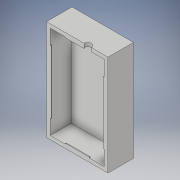
# Autodesk Inventor part: feeder_encolsure
Saved by Autodesk Inventor 2019 (Build 230136000, 136)
## iProperties
Created: 2018-11-21
Part Number: feeder_encolsure
Material: Generic
Document SubType Name: Modeling
Designer: chill
Density: 1 g/cm^3
Appearance: Default
Author: chill
Autodesk Inventor part; units mm, degrees
ref_plane "YZ Plane" through (0, 0, 0) normal (1, 0, 0) x (0, 1, 0)
ref_plane "XZ Plane" through (0, 0, 0) normal (0, 1, 0) x (-1, 0, 0)
ref_plane "XY Plane" through (0, 0, 0) normal (0, 0, 1) x (1, 0, 0)
sketch "Sketch1" plane through (0, 0, 0) normal (0, 0, 1) x (1, 0, 0)
  line L0 (0, 0) -> (36, 0)
  line L1 (36, 0) -> (36, 62)
  line L2 (36, 62) -> (0, 62)
  line L3 (0, 62) -> (0, 0)
  line L4 (-2.5, -2.5) -> (38.5, -2.5)
  line L5 (38.5, -2.5) -> (38.5, 64.5)
  line L6 (38.5, 64.5) -> (-2.5, 64.5)
  line L7 (-2.5, 64.5) -> (-2.5, -2.5)
  dimension "d0" = 36
  dimension "d1" = 62
  dimension "d2" = 2.5
  constraints: 16 end point, 4 parallel, 2 perpendicular, 1 horizontal, 3 other
  measures "d0" distance of L2.end L1.end
  measures "d1" distance of L1.end L0.end
  measures "d2" distance between parallel lines of L3 L7
extrude "Extrusion1" add sketch "Sketch1" along normal blind 17 contours L3 L2 L1 L0 | L7 L6 L5 L4
sketch "Sketch2" plane through (0, 0, 17) normal (0, 0, 1) x (1, 0, 0)
  line L0 (-2.5, -2.5) -> (38.5, -2.5) projected
  line L1 (38.5, -2.5) -> (38.5, 64.5) projected
  line L2 (38.5, 64.5) -> (-2.5, 64.5) projected
  line L3 (-2.5, 64.5) -> (-2.5, -2.5) projected
  line L4 (0, 0) -> (36, 0)
  line L5 (36, 0) -> (36, 62)
  line L6 (36, 62) -> (0, 62)
  line L7 (0, 62) -> (0, 0)
  point P0 (0, 0)
  dimension "d5" = 2.5
  constraints: 8 end point, 3 other
  measures "d5" distance between parallel lines of L3 L7
extrude "Extrusion2" cut sketch "Sketch2" against normal blind 14 contours L7 L6 L5 L4
sketch "Sketch3" plane through (0, 0, 17) normal (0, 0, 1) x (1, 0, 0)
  line L0 (36, 0) -> (0, 0) projected
  line L1 (36, 62) -> (36, 0) projected
  line L2 (0, 62) -> (36, 62) projected
  line L3 (0, 0) -> (0, 62) projected
  line L4 (10, 61.5) -> (26, 61.5)
  line L5 (35.5, 52) -> (35.5, 10)
  line L6 (26, 0.5) -> (10, 0.5)
  line L7 (0.5, 10) -> (0.5, 52)
  line L8 (0, 52) -> (0.5, 52)
  line L9 (35.5, 52) -> (36, 52)
  line L10 (10, 61.5) -> (10, 62)
  line L11 (26, 62) -> (26, 61.5)
  line L12 (36, 10) -> (35.5, 10)
  line L13 (26, 0.5) -> (26, 0)
  line L14 (10, 0) -> (10, 0.5)
  line L15 (0.5, 10) -> (0, 10)
  point P0 (0, 0)
  dimension "d9" = 0.5
  constraints: 24 end point, 8 point on line
  measures "d9" distance between parallel lines of L3 L7
extrude "Extrusion3" add sketch "Sketch3" against normal blind 1 contours L0 L14 L6 L13 | L12 L5 L9 L1 | L3 L8 L7 L15 | L11 L4 L10 L2
fillet "Fillet1" radius 2 4 edges at (0.5, 31, 16) (18, 61.5, 16) (35.5, 31, 16) (18, 0.5, 16)
sketch "Sketch4" plane through (-2.5, 64.5, 0) normal (0, 1, 0) x (1, 0, 0)
  line L0 (41, -17) -> (0, -17) projected
  line L1 (20.5, -17) -> (27.5, -17)
  circle A0 centre (27.5, -17) radius 2.5
  point P0 (2.5, 0)
  dimension "d13" = 7
  dimension "d14" = 5
  constraints: 2 end point, 1 centre point, 1 coincident, 1 midpoint, 1 point on line
  measures "d13" distance of L1.start L1.end
  measures "d14" diameter of A0
extrude "Extrusion4" cut sketch "Sketch4" against normal blind 4
body "Solid1"
